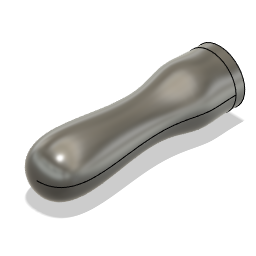
Griff_Feile (Autodesk Fusion 360 design; units mm, degrees)
Autodesk Fusion 360 part; units mm, degrees
sketch "Skizze1" plane through (0, 0, 0) normal (0, 0, 1) x (1, 0, 0)
  circle A0 centre (0, 0) radius 8.75
  dimension "d1" = 17.5
  constraint coincident A0.centre origin
  measures "d1" diameter of A0
extrude "Extrusion1" add sketch "Skizze1" along normal blind 3
sketch "Skizze2" plane through (0, 0, 0) normal (0, 1, 0) x (1, 0, 0)
  line L0 (-8.75, -3) -> (8.75, -3)
  spline S0 degree 5 poles (8.75, -3) (8.75, -3.6089) (8.7713, -4.8074) (8.867, -6.548) (9.0688, -8.7515) (9.1987, -11.3323) (8.979, -13.822) (8.3719, -16.4163) (7.5918, -19.4247) (6.9488, -23.165) (6.7363, -27.8736) (7.1146, -33.6192) (7.9586, -40.1758) (8.8414, -47.0213) (9.1742, -53.4801) (8.2995, -58.8206) (6.142, -61.6598) (3.4944, -62.7563) (1.2455, -63) (0, -63) knots 0 0 0 0 0 0 0.066667 0.133333 0.2 0.266667 0.333333 0.4 0.466667 0.533333 0.6 0.666667 0.733333 0.8 0.866667 0.933333 1 1 1 1 1 1
  line L1 (0, -63) -> (0, -3)
  line L2 (3.5, -63) -> (-3.5, -63)
  line L3 (8.75, 1.4189) -> (8.75, -7.4189)
  point P0 (9, -13)
  point P1 (7, -31)
  dimension "d4" = 60
  dimension "d5" = 7
  dimension "d6" = 9
  dimension "d7" = 7
  dimension "d8" = 10
  dimension "d9" = 28
  constraint coincident L0.end S0.start
  constraint midpoint L0 L1.end
  constraint perpendicular L0 L1
  constraint midpoint S0.end L2
  constraint perpendicular L1 L2
  constraint midpoint L0.end L3
  constraint perpendicular L0 L3
  measures "d4" distance of S0.end L1.end
  measures "d5" distance of P1 L1
  measures "d6" distance of P0 L1
  measures "d7" distance of L2.start L2.end
  measures "d8" distance of L0 P0
  measures "d9" distance of L0 P1
revolve "Drehen1" add sketch "Skizze2" angle 360 about axis through (0, 0, 63) along (0, 0, -1)
sketch "Skizze3" plane through (0, 0, 0) normal (0, 0, -1) x (-1, 0, 0)
  circle A0 centre (0, 0) radius 8.75
  line L0 (-6, 6) -> (6, 6)
  line L1 (6, 6) -> (6, -6)
  line L2 (6, -6) -> (-6, -6)
  line L3 (-6, -6) -> (-6, 6)
  line L4 (-6, 6) -> (6, -6) construction
  line L5 (6, 6) -> (-6, -6) construction
  dimension "d11" = 12
  constraint horizontal L0
  constraint perpendicular L0 L1
  constraint parallel L0 L2
  constraint parallel L1 L3
  constraint coincident L4 A0.centre
  constraint coincident L5 A0.centre
  constraint coincident A0.centre origin
  constraint equal L0 L1
  measures "d11" distance of L1.end L2.end
extrude "Extrusion2" cut sketch "Skizze3" against normal blind 11 contours L0 L1 L2 L3
